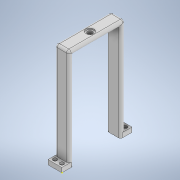
# Autodesk Inventor part: Top clamp for capillary jig - thermal seal - with cam mount
Saved by Autodesk Inventor 2020 (Build 240168000, 168)
## iProperties
Created: 2022-11-27
Part Number: Top clamp for capillary jig - thermal seal - with cam mount
Material: Generic
Document SubType Name: Modeling
Designer: Beaucage
Density: 1 g/cm^3
Appearance: Default
Author: Beaucage
Autodesk Inventor part; units mm, degrees
ref_plane "YZ Plane" through (0, 0, 0) normal (1, 0, 0) x (0, 1, 0)
ref_plane "XZ Plane" through (0, 0, 0) normal (0, 1, 0) x (-1, 0, 0)
ref_plane "XY Plane" through (0, 0, 0) normal (0, 0, 1) x (1, 0, 0)
sketch "Sketch1" plane through (0, 0, 0) normal (0, 1, 0) x (-1, 0, 0)
  line L0 (0, 0) -> (19.05, 0)
  line L1 (19.05, 0) -> (19.05, -9.525)
  line L2 (19.05, -9.525) -> (0, -9.525)
  line L3 (0, -9.525) -> (0, 0)
  line L4 (0, -9.525) -> (0, -86.995)
  line L5 (0, -9.525) -> (77.47, -9.525) construction
  line L6 (0, -86.995) -> (19.05, -86.995)
  line L7 (19.05, -86.995) -> (19.05, -96.52)
  line L8 (19.05, -96.52) -> (0, -96.52)
  line L9 (0, -96.52) -> (0, -86.995)
  dimension "d0" = 19.05
  dimension "d1" = 9.525
  dimension "d23" = 77.47
  dimension "d24" = 90
  dimension "d25" = 19.05
  dimension "d26" = 9.525
  constraints: 20 end point, 4 parallel, 3 horizontal, 3 perpendicular, 1 vertical
  measures "d0" distance of L1.end L2.end
  measures "d1" distance of L0.end L1.end
  measures "d23" distance of L2.end L4.end
  measures "d24" angle of L4 L5
  measures "d25" distance of L7.end L8.end
  measures "d26" distance of L6.end L7.end
extrude "Extrusion1" add sketch "Sketch1" along normal blind 6.35
sketch "Sketch2" plane through (-19.05, 0, 0) normal (0, 0, 1) x (1, 0, 0)
  line L0 (19.05, 0) -> (0, 0) projected
  point P0 (9.525, 0)
  constraints: 1 midpoint
hole "Hole1" at (-9.525, 0, 0) direction (0, 0, -1) diameter 1.5 end through all
sketch "Sketch3" plane through (0, 6.35, 0) normal (0, 1, 0) x (1, 0, 0)
  line L0 (-19.05, 0) -> (-10.275, 0) projected
  line L1 (-19.05, 0) -> (-14.2748, 0)
  line L2 (-14.2748, 0) -> (-14.2748, 4.7752)
  line L3 (-14.2748, 4.7752) -> (-19.05, 4.7752)
  line L4 (-19.05, 4.7752) -> (-19.05, 0)
  line L5 (-19.05, 0) -> (0, 0) projected
  line L6 (0, 0) -> (-4.7752, 0)
  line L7 (-4.7752, 0) -> (-4.7752, 4.7752)
  line L8 (-4.7752, 4.7752) -> (0, 4.7752)
  line L9 (0, 4.7752) -> (0, 0)
  line L10 (-19.05, 96.52) -> (-14.2748, 96.52)
  line L11 (-14.2748, 96.52) -> (-14.2748, 91.7448)
  line L12 (-14.2748, 91.7448) -> (-19.05, 91.7448)
  line L13 (-19.05, 91.7448) -> (-19.05, 96.52)
  line L14 (0, 96.52) -> (-8.775, 96.52) projected
  line L15 (0, 96.52) -> (-4.7752, 96.52)
  line L16 (-4.7752, 96.52) -> (-4.7752, 91.7448)
  line L17 (-4.7752, 91.7448) -> (0, 91.7448)
  line L18 (0, 91.7448) -> (0, 96.52)
  dimension "d11" = 4.7752
  dimension "d12" = 4.7752
  dimension "d13" = 4.7752
  dimension "d14" = 4.7752
  dimension "d27" = 4.7752
  dimension "d28" = 4.7752
  dimension "d29" = 4.7752
  constraints: 32 end point, 8 parallel, 4 horizontal, 4 perpendicular
  measures "d11" distance of L3.end L2.end
  measures "d12" distance of L2.end L1.end
  measures "d13" distance of L7.end L8.end
  measures "d14" distance of L6.end L7.end
  measures "d27" distance of L10.end L11.end
  measures "d28" distance of L17.end L16.end
  measures "d29" distance of L16.end L15.end
hole "Hole2" at (-14.2748, 6.35, -4.7752) at (-4.7752, 6.35, -4.7752) at (-14.2748, 6.35, -91.7448) at (-4.7752, 6.35, -91.7448) direction (0, -1, 0) diameter 3.2766 end through all counterbore diameter 5.5626 counterbore depth 2.8448 clearance for "Socket Head Cap Screw" size "#4" standard "Ansi Unified Screw Threads"
sketch "Sketch4" plane through (0, 0, 0) normal (1, 0, 0) x (0, 0, -1)
  point P0 (0, 0)
sketch "Sketch5" plane through (-19.05, 6.35, -86.995) normal (0, 0, 1) x (1, 0, 0)
  arc A0 (10.275, -6.35) -> (8.775, -6.35) centre (9.525, -6.35) ccw projected
  line L0 (10.275, -6.35) -> (19.05, -6.35) projected
  line L1 (19.05, -6.35) -> (19.05, 0) projected
  line L2 (0, 0) -> (19.05, 0) projected
  line L3 (0, -6.35) -> (0, 0) projected
  line L4 (0, -6.35) -> (8.775, -6.35) projected
extrude "Extrusion2" add sketch "Sketch5" along normal blind 6.35
sketch "Sketch6" plane through (0, 6.35, -9.525) normal (0, 0, -1) x (-1, 0, 0)
  arc A0 (10.275, -6.35) -> (8.775, -6.35) centre (9.525, -6.35) ccw projected
  line L0 (10.275, -6.35) -> (19.05, -6.35) projected
  line L1 (19.05, -6.35) -> (19.05, 0) projected
  line L2 (0, 0) -> (19.05, 0) projected
  line L3 (0, -6.35) -> (0, 0) projected
  line L4 (0, -6.35) -> (8.775, -6.35) projected
extrude "Extrusion3" add sketch "Sketch6" along normal blind 6.35
sketch "Sketch7" plane through (0, 6.35, 0) normal (0, 1, 0) x (1, 0, 0)
  line L0 (-19.05, 15.875) -> (0, 15.875) projected
  line L1 (0, 0) -> (0, 15.875) projected
  line L2 (-19.05, 15.875) -> (0, 15.875)
  line L3 (0, 15.875) -> (0, 9.525)
  line L4 (0, 9.525) -> (-19.05, 9.525)
  line L5 (-19.05, 9.525) -> (-19.05, 15.875)
  line L6 (-19.05, 96.52) -> (-19.05, 80.645) projected
  line L7 (0, 96.52) -> (0, 80.645) projected
  line L8 (-19.05, 80.645) -> (0, 80.645)
  line L9 (0, 80.645) -> (0, 86.995)
  line L10 (0, 86.995) -> (-19.05, 86.995)
  line L11 (-19.05, 86.995) -> (-19.05, 80.645)
  dimension "d34" = 6.35
  dimension "d35" = 6.35
  constraints: 16 end point, 4 parallel, 2 horizontal, 2 perpendicular, 2 point on line
  measures "d34" distance of L2.end L3.end
  measures "d35" distance of L9.end L8.end
extrude "Extrusion4" add sketch "Sketch7" along normal blind 127
sketch "Sketch8" plane through (0, 133.35, 0) normal (0, 1, 0) x (1, 0, 0)
  line L0 (-19.05, 9.525) -> (0, 9.525) projected
  line L1 (0, 80.645) -> (0, 86.995) projected
  line L2 (-19.05, 9.525) -> (0, 9.525)
  line L3 (0, 9.525) -> (0, 86.995)
  line L4 (0, 86.995) -> (-19.05, 86.995)
  line L5 (-19.05, 86.995) -> (-19.05, 9.525)
  point P0 (0, 0)
  constraints: 8 end point, 2 parallel, 1 horizontal, 1 perpendicular
extrude "Extrusion5" add sketch "Sketch8" along normal blind 6.35
sketch "Sketch9" plane through (0, 139.7, 0) normal (0, 1, 0) x (1, 0, 0)
  line L0 (0, 9.525) -> (0, 86.995) projected
  line L1 (0, 86.995) -> (-19.05, 86.995) projected
  line L2 (-19.05, 86.995) -> (-19.05, 9.525) projected
  line L3 (-19.05, 9.525) -> (0, 9.525) projected
  point P0 (0, 0)
  point P1 (-9.525, 48.26)
hole "Hole3" at (-9.525, 139.7, -48.26) direction (0, -1, 0) diameter 6.7564 end through all counterbore diameter 11.1252 counterbore depth 1.5875 clearance for "Socket Head Cap Screw" size "1/4" standard "Ansi Unified Screw Threads"
fillet "Fillet2" radius 3.175 14 edges at (0, 66.675, -15.875) (0, 73.025, -9.525) (0, 133.35, -48.26) (0, 139.7, -48.26) (-19.05, 139.7, -48.26) (-9.525, 139.7, -9.525) (-19.05, 73.025, -9.525) (-9.525, 139.7, -86.995) (0, 73.025, -86.995) (0, 66.675, -80.645) (-19.05, 66.675, -80.645) (-19.05, 73.025, -86.995) (-19.05, 133.35, -48.26) (-19.05, 66.675, -15.875)
body "Solid1"
